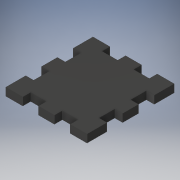
# Autodesk Inventor part: right
Saved by Autodesk Inventor 2019 (Build 230136000, 136)
## iProperties
Created: 2018-06-06
Part Number: right
Material: PBT Plastic Black
Document SubType Name: Modeling
Designer: stra92745
Density: 1.31 g/cm^3
Appearance: Smooth - White
Author: stra92745
Autodesk Inventor part; units mm, degrees
ref_plane "YZ Plane" through (0, 0, 0) normal (1, 0, 0) x (0, 1, 0)
ref_plane "XZ Plane" through (0, 0, 0) normal (0, 1, 0) x (-1, 0, 0)
ref_plane "XY Plane" through (0, 0, 0) normal (0, 0, 1) x (1, 0, 0)
sketch "Sketch1" plane through (0, 0, 0) normal (0, 1, 0) x (-1, 0, 0)
  line L0 (0, 0) -> (-41, 0)
  line L1 (-41, 0) -> (-41, -44)
  line L2 (-41, -44) -> (0, -44)
  line L3 (0, -44) -> (0, 0)
  dimension "d0" = 41
  dimension "d1" = 44
  constraints: 8 end point, 2 parallel, 1 horizontal, 1 perpendicular
  measures "d0" distance of L2.end L1.end
  measures "d1" distance of L1.end L0.end
extrude "Extrusion1" add sketch "Sketch1" along normal blind 4
sketch "Sketch2" plane through (0, 4, 0) normal (0, 1, 0) x (1, 0, 0)
  line L0 (41, 44) -> (0, 44) construction
  line L1 (0, 44) -> (0, 0) construction
  line L2 (0, 0) -> (41, 0) construction
  line L3 (41, 0) -> (41, 44) construction
  line L4 (4, 4) -> (4, 40) construction
  line L5 (4, 40) -> (37, 40) construction
  line L6 (37, 40) -> (37, 4) construction
  line L7 (37, 4) -> (4, 4) construction
  line L8 (0, 34) -> (4, 34)
  line L9 (4, 34) -> (4, 26)
  line L10 (4, 26) -> (0, 26)
  line L11 (0, 34) -> (0, 26)
  line L12 (0, 22) -> (41, 22) construction
  line L13 (20.5, 0) -> (20.5, 44) construction
  line L14 (41, 44) -> (0, 44) construction
  line L15 (8.5, 44) -> (8.5, 40)
  line L16 (8.5, 40) -> (16.5, 40)
  line L17 (16.5, 40) -> (16.5, 44)
  line L18 (16.5, 44) -> (8.5, 44)
  line L19 (41, 34) -> (37, 34)
  line L20 (37, 34) -> (37, 26)
  line L21 (37, 26) -> (41, 26)
  line L22 (41, 34) -> (41, 26)
  line L23 (32.5, 44) -> (32.5, 40)
  line L24 (32.5, 40) -> (24.5, 40)
  line L25 (24.5, 40) -> (24.5, 44)
  line L26 (24.5, 44) -> (32.5, 44)
  line L27 (41, 0) -> (0, 0)
  line L28 (4, 4) -> (37, 4)
  line L29 (0, 10) -> (4, 10)
  line L30 (4, 10) -> (4, 18)
  line L31 (4, 18) -> (0, 18)
  line L32 (0, 10) -> (0, 18)
  line L33 (41, 0) -> (0, 0)
  line L34 (8.5, 0) -> (8.5, 4)
  line L35 (8.5, 4) -> (16.5, 4)
  line L36 (16.5, 4) -> (16.5, 0)
  line L37 (16.5, 0) -> (8.5, 0)
  line L38 (24.5, 4) -> (24.5, 0)
  line L39 (32.5, 0) -> (32.5, 4)
  line L40 (37, 10) -> (37, 18)
  line L41 (41, 10) -> (37, 10)
  line L42 (41, 10) -> (41, 18)
  line L43 (37, 18) -> (41, 18)
  line L44 (24.5, 0) -> (32.5, 0)
  line L45 (32.5, 4) -> (24.5, 4)
  dimension "d8" = 4
  dimension "d9" = 8
  dimension "d10" = 4
  dimension "d11" = 8
  dimension "d12" = 4
  constraints: 82 end point, 24 symmetric about line, 12 point on line, 4 midpoint, 4 perpendicular, 2 collinear, 3 other
  measures "d8" distance between parallel lines of L1 L4
  measures "d9" distance of L8.end L9.end
  measures "d10" distance between parallel lines of L12 L10
  measures "d11" distance of L15.end L16.end
  measures "d12" distance between parallel lines of L13 L17
extrude "Extrusion2" cut sketch "Sketch2" against normal up to surface (4 mm away) contours L8 L9 L10 L11 | L18 L17 L16 L15 | L22 L21 L20 L19 | L23 L24 L25 L26 | L27 L38 L28 L39 | L27 L34 L28 L36 | L32 L31 L30 L29 | L40 L43 L42 L41
body "Solid1"
